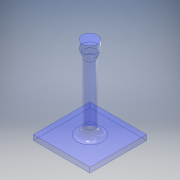
# Autodesk Inventor part: Base
Saved by Autodesk Inventor 2017 (Build 210142000, 142)
## iProperties
Created: 2021-02-24
Part Number: Base
Material: Generic
Document SubType Name: Modeling
Designer: Lenovo Y900
Density: 1 g/cm^3
Appearance: Clear - Blue
Author: Lenovo Y900
Autodesk Inventor part; units mm, degrees
ref_plane "YZ Plane" through (0, 0, 0) normal (1, 0, 0) x (0, 1, 0)
ref_plane "XZ Plane" through (0, 0, 0) normal (0, 1, 0) x (-1, 0, 0)
ref_plane "XY Plane" through (0, 0, 0) normal (0, 0, 1) x (1, 0, 0)
sketch "Sketch1" plane through (0, 0, 0) normal (0, 0, 1) x (1, 0, 0)
  circle A0 centre (0, 0) radius 5
  dimension "d0" = 10
  constraints: 1 centre point, 1 coincident
  measures "d0" diameter of A0
extrude "Extrusion1" add sketch "Sketch1" along normal blind 70
sketch "Sketch2" plane through (0, 0, 70) normal (0, 0, 1) x (1, 0, 0)
  circle A0 centre (0, 0) radius 7.5
  dimension "d3" = 15
  constraints: 1 centre point, 1 coincident
  measures "d3" diameter of A0
extrude "Extrusion2" add sketch "Sketch2" along normal blind 10
fillet "Fillet1" radius 7.25 2 edges at (-5, 0, 70) (-7.5, 0, 70)
sketch "Sketch3" plane through (0, 0, 0) normal (0, 0, -1) x (-1, 0, 0)
  line L0 (27.5, -27.5) -> (-27.5, -27.5)
  line L1 (-27.5, -27.5) -> (-27.5, 27.5)
  line L2 (-27.5, 27.5) -> (27.5, 27.5)
  line L3 (27.5, 27.5) -> (27.5, -27.5)
  line L4 (27.5, -27.5) -> (-27.5, 27.5) construction
  line L5 (-27.5, -27.5) -> (27.5, 27.5) construction
  point P0 (0, 0)
  dimension "d7" = 55
  dimension "d8" = 55
  constraints: 12 end point, 2 midpoint, 2 parallel, 1 horizontal, 1 perpendicular
  measures "d7" distance of L1.end L2.end
  measures "d8" distance of L0.end L1.end
extrude "Extrusion3" add sketch "Sketch3" along normal blind 5
fillet "Fillet2" radius 7.25 1 edges at (-5, 0, 0)
body "Solid1"
